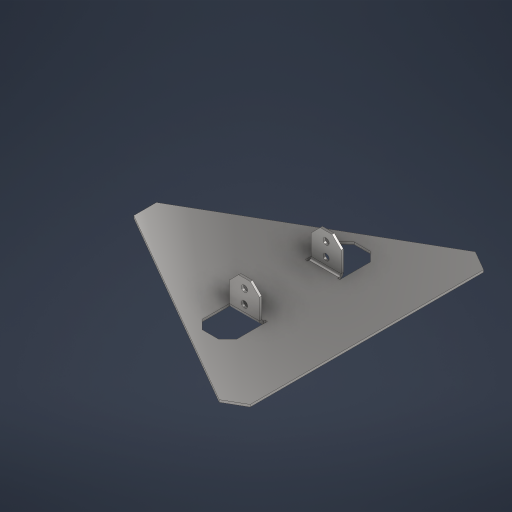
# Autodesk Inventor part: BasePlate
Saved by Autodesk Inventor 2023 (Build 270158000, 158)
## iProperties
Created: 2023-02-24
Part Number: BasePlate
Material: Stainless Steel
Document SubType Name: Sheet Metal
Designer: roota
Density: 8 g/cm^3
Sheet Metal Rule: Default_mm
Appearance: Semi-Polished
Mass: 400.897 g
Surface Area: 523.871 cm^2
Volume: 50.1121 cm^3
Author: roota
Autodesk Inventor part; units mm, degrees
ref_plane "YZ Plane" through (0, 0, 0) normal (1, 0, 0) x (0, 1, 0)
ref_plane "XZ Plane" through (0, 0, 0) normal (0, 1, 0) x (-1, 0, 0)
ref_plane "XY Plane" through (0, 0, 0) normal (0, 0, 1) x (1, 0, 0)
sketch "Sketch1" plane through (0, 0, 0) normal (0, 1, 0) x (-1, 0, 0)
  line L0 (124.5994, -10) -> (-53.6394, -112.9062)
  line L1 (-70.9599, -102.9062) -> (-70.9599, 102.9062)
  line L2 (-53.6394, 112.9062) -> (124.5994, 10)
  circle A0 centre (0, 0) radius 70.9599 construction
  line L3 (124.5994, 10) -> (124.5994, -10)
  line L4 (-53.6394, -112.9062) -> (-70.9599, -102.9062)
  line L5 (-70.9599, 102.9062) -> (-53.6394, 112.9062)
  circle A1 centre (0, 0) radius 125 construction
  point P0 (141.9199, 0)
  point P1 (-70.9599, -122.9062)
  point P2 (-70.9599, 122.9062)
  dimension "d7" = 250
  dimension "d1" = 20
  dimension "d2" = 20
  dimension "d3" = 20
  dimension "d4" = 20
  dimension "d5" = 20
  dimension "d6" = 20
  measures "d1" distance of L2.end point (141.92, 0)
  measures "d2" distance of L0.start point (141.92, 0)
  measures "d3" distance of L0.end point (-70.96, -122.906)
  measures "d4" distance of L1.start point (-70.96, -122.906)
  measures "d5" distance of L1.end point (-70.96, 122.906)
  measures "d6" distance of L2.start point (-70.96, 122.906)
extrude "Plate1" add sketch "Sketch1" along normal blind 2
sketch "Sketch2" plane through (0, 2, 0) normal (0, 1, 0) x (1, 0, 0)
  circle A0 centre (0, 0) radius 40 construction
  line L0 (15.1987, 37) -> (-15.1987, 37)
  line L1 (-15.1987, 37) -> (-15.1987, 57.3146)
  line L2 (0.2732, 67) -> (10.6706, 67)
  line L3 (15.1987, 57.3127) -> (15.1987, 37)
  line L4 (15.1987, -37) -> (-15.1987, -37)
  line L5 (-15.1987, -37) -> (-15.1987, -57.3146)
  line L6 (0.2732, -67) -> (10.6706, -67)
  line L7 (15.1987, -57.3127) -> (15.1987, -37)
  line L8 (-15.1987, 57.3146) -> (-15.1987, 67)
  line L9 (-15.1987, 67) -> (0.2732, 67)
  line L10 (10.6706, 67) -> (15.1987, 67)
  line L11 (15.1987, 67) -> (15.1987, 57.3127)
  line L12 (0.2732, -67) -> (-15.1987, -67)
  line L13 (-15.1987, -57.3146) -> (-15.1987, -67)
  line L14 (10.6706, -67) -> (15.1987, -67)
  line L15 (15.1987, -67) -> (15.1987, -57.3127)
  circle A1 centre (0, 0) radius 70.9599 construction
  line L16 (-124.5994, 10) -> (53.6394, 112.9062) projected
  line L17 (70.9599, 102.9062) -> (70.9599, -102.9062) projected
  point P0 (0, 0)
  dimension "d9" = 80
  dimension "d10" = 74
  dimension "d11" = 30
  constraints: 32 end point, 9 point on line, 6 perpendicular, 4 equal length, 4 horizontal, 4 parallel, 3 point on circle, 2 centre point, 2 coincident, 2 tangent, 1 vertical
  measures "d9" diameter of A0
  measures "d10" distance between parallel lines of L0 L4
  measures "d11" distance of L10.end L0.start
extrude "Cut1" cut sketch "Sketch2" against normal blind 2
sketch "Sketch3" plane through (15.1987, 0, 35) normal (0, 0, 1) x (1, 0, 0)
  line L0 (-28.3974, 0) -> (-2, 0)
  line L1 (-2, 0) -> (-2, 30)
  line L2 (-2, 30) -> (-28.3974, 30)
  line L3 (-28.3974, 30) -> (-28.3974, 0)
  constraints: 8 end point
edge flange "Flange1" height 30 angle 90 thickness 2 bend radius 2 thickness toward (0, 0, 1) relief straight relief width 2 relief depth 1 corner gap 2 corner form 0 edges at (0, 2, 37) (0, 2, -37) wall of the first edge with corners at (-13.1987, 0, 35) (13.1987, 0, 35) (13.1987, 30, 35) (-13.1987, 30, 35)
bend "Bend1"
corner "Corner1"
chamfer "Corner Chamfer1" distance 8 angle 45 8 edges at (13.1987, 30, 36) (-13.1987, 30, 36) (13.1987, 30, -36) (-13.1987, 30, -36) (15.1987, 1, 67) (-15.1987, 1, 67) (-15.1987, 1, -67) (15.1987, 1, -67)
sketch "Sketch4" plane through (-13.1987, 4, 37) normal (0, 0, 1) x (1, 0, 0)
  circle A0 centre (13.1987, 6) radius 2.75
  circle A1 centre (13.1987, 18) radius 2.75
  line L0 (66.8381, -2) -> (-111.4007, -2) projected
  line L1 (0, 0) -> (0, 18) projected
  line L2 (26.3974, 18) -> (26.3974, 0) projected
  point P0 (13.1987, -4)
  dimension "d35" = 5.5
  dimension "d36" = 12
  dimension "d37" = 8
  dimension "d39" = 26.3974
  dimension "d40" = 13.1987
  constraints: 2 centre point, 1 equal radius, 1 vertical alignment
  measures "d35" diameter of A1
  measures "d36" distance of A1.centre A0.centre
  measures "d37" distance from line of L0 A0.centre
  measures "d39" distance between parallel lines of L1 L2
  measures "d40" distance from line of A1.centre L1
extrude "Extrusion1" cut sketch "Sketch4" against normal through all
equation "\"d20\" = Thickness"
equation "\"d40\" = 0.5 * d39"
equation "\"d8\" = Thickness"
equation "\"d22\" = BendReliefWidth"
equation "\"d23\" = BendReliefDepth"
equation "\"d24\" = MinimumRemnant"
equation "\"d25\" = TransitionRadius"
equation "\"d26\" = d11"
equation "\"d28\" = BendRadius"
equation "\"d29\" = CornerReliefSize"
equation "\"d30\" = GapSize"
equation "\"d31\" = JacobiRadiusSize"
equation "\"d2\" = d1"
equation "\"d3\" = d1"
equation "\"d4\" = d3"
equation "\"d5\" = d1"
equation "\"d6\" = d5"
equation "\"BendRadius\" = Thickness"
equation "\"BendReliefWidth\" = Thickness"
equation "\"BendReliefDepth\" = 0.5 * Thickness"
equation "\"CornerReliefSize\" = 4 * Thickness"
equation "\"MinimumRemnant\" = 2 * Thickness"
equation "\"TransitionRadius\" = BendRadius"
equation "\"JacobiRadiusSize\" = BendRadius"
equation "\"GapSize\" = Thickness"
equation "\"Thickness\" = 2"
body "Solid1"
